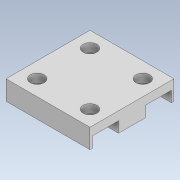
# Autodesk Inventor part: INTERFACE_MANIFOLD_KORK
Saved by Autodesk Inventor 2020 (Build 240168000, 168)
## iProperties
Created: 2020-07-07
Part Number: INTERFACE_MANIFOLD_KORK
Material: Generic
Document SubType Name: Modeling
Designer: Admin
Density: 1 g/cm^3
Appearance: Default
Author: Admin
Autodesk Inventor part; units mm, degrees
ref_plane "YZ Plane" through (0, 0, 0) normal (1, 0, 0) x (0, 1, 0)
ref_plane "XZ Plane" through (0, 0, 0) normal (0, 1, 0) x (-1, 0, 0)
ref_plane "XY Plane" through (0, 0, 0) normal (0, 0, 1) x (1, 0, 0)
sketch "Sketch1" plane through (0, 0, 0) normal (0, 1, 0) x (-1, 0, 0)
  line L0 (0, 0) -> (19.4, 0)
  line L1 (19.4, 0) -> (19.4, -19.4)
  line L2 (19.4, -19.4) -> (0, -19.4)
  line L3 (0, -19.4) -> (0, 0)
  dimension "d0" = 19.4
  dimension "d1" = 19.4
  constraints: 8 end point, 2 parallel, 1 horizontal, 1 perpendicular
  measures "d0" distance of L0.start L0.end
  measures "d1" distance of L2.end L0.start
extrude "Extrusion1" add sketch "Sketch1" along normal blind 4.5
sketch "Sketch2" plane through (0, 4.5, 0) normal (0, 1, 0) x (1, 0, 0)
  circle A0 centre (-3.6, 3.6) radius 1.6
  line L0 (-19.4, 0) -> (0, 0) projected
  line L1 (0, 0) -> (0, 19.4) projected
  dimension "d4" = 3.2
  dimension "d5" = 3.6
  dimension "d6" = 3.6
  constraints: 1 centre point
  measures "d4" diameter of A0
  measures "d5" distance from line of L0 A0.centre
  measures "d6" distance from line of L1 A0.centre
extrude "Extrusion2" cut sketch "Sketch2" against normal through all
pattern_linear "Rectangular Pattern1" count 2 spacing 12.2 along (0, 0, -1) count 2 spacing 12.2 along (-1, 0, 0) of "Extrusion2"
sketch "Sketch3" plane through (0, 0, 0) normal (1, 0, 0) x (0, 0, -1)
  line L0 (0.6, 2.5) -> (6.6, 2.5)
  line L1 (6.6, 2.5) -> (6.6, 0)
  line L2 (6.6, 0) -> (0.6, 0)
  line L3 (0.6, 0) -> (0.6, 2.5)
  line L4 (0, 0) -> (0, 4.5) projected
  line L5 (0, 0) -> (19.4, 0) projected
  line L6 (12.8, 2.5) -> (18.8, 2.5)
  line L7 (18.8, 2.5) -> (18.8, 0)
  line L8 (18.8, 0) -> (12.8, 0)
  line L9 (12.8, 0) -> (12.8, 2.5)
  line L10 (19.4, 0) -> (19.4, 4.5) projected
  dimension "d15" = 6
  dimension "d16" = 2.5
  dimension "d17" = 0.6
  dimension "d18" = 6
  dimension "d19" = 2.5
  dimension "d20" = 0.6
  constraints: 16 end point, 4 parallel, 2 horizontal, 2 perpendicular, 2 point on line
  measures "d15" distance of L0.start L0.end
  measures "d16" distance of L2.end L0.start
  measures "d17" distance between parallel lines of L4 L3
  measures "d18" distance of L6.start L6.end
  measures "d19" distance of L8.end L6.start
  measures "d20" distance between parallel lines of L10 L7
extrude "Extrusion3" cut sketch "Sketch3" against normal through all
body "Solid1"
